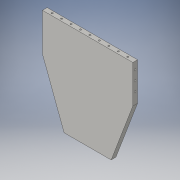
# Autodesk Inventor part: top
Saved by Autodesk Inventor 2016 (Build 200138000, 138)
## iProperties
Created: 2015-09-30
Part Number: top
Material: Generic
Document SubType Name: Modeling
Designer: Jesse Stevenson
Density: 1 g/cm^3
Appearance: Default
Author: Jesse Stevenson
Autodesk Inventor part; units mm, degrees
ref_plane "YZ Plane" through (0, 0, 0) normal (1, 0, 0) x (0, 1, 0)
ref_plane "XZ Plane" through (0, 0, 0) normal (0, 1, 0) x (-1, 0, 0)
sketch "Sketch1" plane through (0, 0, 0) normal (0, 0, 1) x (1, 0, 0)
  line L0 (29.0703, 0) -> (121.3612, 0)
  line L1 (121.3612, 0) -> (121.3612, 127.9398)
  line L2 (121.3612, 127.9398) -> (0, 127.9398)
  line L3 (0, 127.9398) -> (0, 13.0299)
  line L4 (0, 77.1398) -> (121.3612, 77.1398) construction
  line L5 (29.0703, 0) -> (29.0703, 26.0597) construction
  line L6 (92.2909, 0) -> (92.2909, 26.0597) construction
  line L7 (29.0703, 13.0299) -> (0, 13.0299) construction
  line L8 (92.2909, 13.0299) -> (121.3612, 13.0299) construction
  line L9 (0, 77.1398) -> (29.0703, 0)
  line L10 (92.2909, 0) -> (121.3612, 77.1398)
  point P0 (0, 0)
  dimension "d0" = 121.3612
  dimension "d1" = 127.9398
  dimension "d2" = 50.8
  dimension "d3" = 63.2206
  constraints: 22 end point, 5 point on line, 3 perpendicular, 2 midpoint, 2 parallel, 2 vertical, 1 collinear, 1 horizontal
  measures "d0" distance of L2.end L1.end
  measures "d1" distance of L0.end L1.end
  measures "d2" distance between parallel lines of L4 L2
  measures "d3" distance between parallel lines of L6 L5
extrude "Extrusion1" add sketch "Sketch1" along normal blind 6.35 contours L9 L3 L2 L1 L10 L0
sketch "Sketch2" plane through (0, 127.9398, 0) normal (0, 1, 0) x (1, 0, 0)
  line L0 (121.3612, 0) -> (0, 0) construction
  line L1 (0, 0) -> (0, -6.35) construction
  line L2 (121.3612, -6.35) -> (0, -6.35) construction
  line L3 (121.3612, 0) -> (121.3612, -6.35) construction
  line L4 (121.3612, -6.35) -> (0, -6.35) construction
  line L5 (60.6806, -6.35) -> (60.6806, 0) construction
  line L6 (121.3612, 0) -> (0, 0) construction
  circle A0 centre (60.6806, -3.175) radius 1.0541
  circle A1 centre (47.9806, -3.175) radius 1.0541
  circle A2 centre (35.2806, -3.175) radius 1.0541
  circle A3 centre (22.5806, -3.175) radius 1.0541
  circle A4 centre (9.8806, -3.175) radius 1.0541
  circle A5 centre (60.6806, -3.175) radius 1.0541
  circle A6 centre (73.3806, -3.175) radius 1.0541
  circle A7 centre (86.0806, -3.175) radius 1.0541
  circle A8 centre (98.7806, -3.175) radius 1.0541
  circle A9 centre (111.4806, -3.175) radius 1.0541
  dimension "d6" = 2.1082
  dimension "d9" = 12.7
  constraints: 10 centre point, 4 symmetric about line, 3 midpoint, 2 end point, 1 horizontal, 13 other
  measures "d6" diameter of A0
  measures "d9" distance of A0.centre A1.centre
extrude "Extrusion2" cut sketch "Sketch2" against normal blind 3.6322
sketch "Sketch3" plane through (121.3612, 77.1398, 0) normal (1, 0, 0) x (0, 0, -1)
  line L0 (0, 0) -> (0, 50.8) construction
  line L1 (0, 50.8) -> (-6.35, 50.8) construction
  line L2 (-6.35, 0) -> (-6.35, 50.8) construction
  line L3 (0, 0) -> (-6.35, 0) construction
  line L4 (0, 50.8) -> (-6.35, 50.8) construction
  line L5 (-3.175, 50.8) -> (-3.175, 0) construction
  line L6 (0, 0) -> (-6.35, 0) construction
  circle A0 centre (-3.175, 40.9194) radius 1.0541
  point P0 (0, -77.1398)
  dimension "d16" = 2.1082
  dimension "d17" = 9.8806
  constraints: 2 end point, 2 midpoint, 1 centre point, 1 point on line
  measures "d16" diameter of A0
  measures "d17" distance from line of L1 A0.centre
extrude "Extrusion3" cut sketch "Sketch3" against normal blind 25.4
pattern_linear "Rectangular Pattern1" count 3 spacing 12.7 along (0, -1, 0) of "Extrusion3"
ref_plane "Work Plane1" through (60.6806, 127.9398, 0) normal (1, 0, 0) x (0, 0, 1)
mirror "Mirror1" about plane through (60.6806, 127.9398, 0) normal (1, 0, 0) of "Extrusion3", "Rectangular Pattern1"
body "Solid1"
